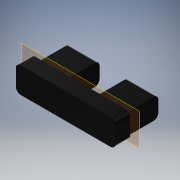
# Autodesk Inventor part: Holster_Button
Saved by Autodesk Inventor 2018 (Build 220112000, 112)
## iProperties
Created: 2018-02-02
Part Number: Holster_Button
Material: Generic
Document SubType Name: Modeling
Designer: Mandus
Density: 1 g/cm^3
Appearance: Default
Author: Mandus
Autodesk Inventor part; units mm, degrees
ref_plane "YZ Plane" through (0, 0, 0) normal (1, 0, 0) x (0, 1, 0)
ref_plane "XZ Plane" through (0, 0, 0) normal (0, 1, 0) x (-1, 0, 0)
ref_plane "XY Plane" through (0, 0, 0) normal (0, 0, 1) x (1, 0, 0)
ref_plane "Work Plane1" through (1.1136, 1.5, 0.2896) normal (0, -1, 0) x (1, 0, 0)
sketch "Sketch3" plane through (1.1136, 1.5, 0.2896) normal (0, -1, 0) x (1, 0, 0)
  line L0 (-8.5, 0) -> (-8.5, 5) construction
  line L1 (-8.5, 5) -> (-1.5, 5) construction
  line L2 (-1.5, 5) -> (-1.5, 0) construction
  line L3 (0, 0) -> (-1.5, 0) construction
  line L4 (0, 0) -> (0, 6) construction
  line L5 (0, 6) -> (-22.065, 6) construction
  line L6 (-22.065, 0) -> (-22.065, 6) construction
  line L7 (-20.565, 0) -> (-22.065, 0) construction
  line L8 (-20.565, 0) -> (-20.565, 5) construction
  line L9 (-20.565, 5) -> (-13.565, 5) construction
  line L10 (-13.565, 5) -> (-13.565, 0) construction
  line L11 (-8.5, 0) -> (-13.565, 0) construction
  line L12 (-0.8, 0) -> (-21.265, 0)
  line L13 (-21.265, 0) -> (-21.265, 5.3)
  line L14 (-21.265, 5.3) -> (-0.8, 5.3)
  line L15 (-0.8, 5.3) -> (-0.8, 0)
  point P0 (-1.1136, -0.2896)
  dimension "d26" = 0.8
  dimension "d27" = 0.8
  dimension "d28" = 0.7
  constraints: 8 end point, 2 parallel, 1 horizontal, 1 perpendicular, 1 point on line
  measures "d26" distance from line of L4 L14.end
  measures "d27" distance from line of L6 L13.end
  measures "d28" distance from line of L5 L13.end
extrude "Extrusion3" add sketch "Sketch3" along normal blind 3
sketch "Sketch4" plane through (1.1136, 1.5, 0.2896) normal (0, 1, 0) x (1, 0, 0)
  line L0 (-8.5, 0) -> (-8.5, -5) construction
  line L1 (-8.5, -5) -> (-1.5, -5) construction
  line L2 (-1.5, -5) -> (-1.5, 0) construction
  line L3 (0, 0) -> (-1.5, 0) construction
  line L4 (0, 0) -> (0, -6) construction
  line L5 (0, -6) -> (-22.065, -6) construction
  line L6 (-22.065, 0) -> (-22.065, -6) construction
  line L7 (-20.565, 0) -> (-22.065, 0) construction
  line L8 (-20.565, 0) -> (-20.565, -5) construction
  line L9 (-20.565, -5) -> (-13.565, -5) construction
  line L10 (-13.565, -5) -> (-13.565, 0) construction
  line L11 (-8.5, 0) -> (-13.565, 0) construction
  line L12 (-2, 0) -> (-8, 0)
  line L13 (-8, 0) -> (-8, -4.3)
  line L14 (-8, -4.3) -> (-2, -4.3)
  line L15 (-2, -4.3) -> (-2, 0)
  line L16 (-0.8, 0) -> (-21.265, 0) projected
  line L17 (-14.065, 0) -> (-20.065, 0)
  line L18 (-20.065, 0) -> (-20.065, -4.3)
  line L19 (-20.065, -4.3) -> (-14.065, -4.3)
  line L20 (-14.065, -4.3) -> (-14.065, 0)
  point P0 (-1.1136, 0.2896)
  point P1 (-5, 0)
  point P2 (-11.0325, 0)
  dimension "d31" = 0.5
  dimension "d32" = 0.5
  dimension "d33" = 0.7
  dimension "d34" = 0.7
  dimension "d35" = 0.5
  dimension "d36" = 0.5
  constraints: 16 end point, 4 parallel, 2 horizontal, 2 midpoint, 2 perpendicular, 1 horizontal alignment, 2 other
  measures "d31" distance from line of L0 L13.end
  measures "d32" distance from line of L2 L14.end
  measures "d33" distance from line of L1 L14.end
  measures "d34" distance from line of L9 L19.end
  measures "d35" distance from line of L10 L19.end
  measures "d36" distance from line of L8 L18.end
extrude "Extrusion4" add sketch "Sketch4" along normal blind 7
fillet "Fillet6" radius 1 4 edges at (-20.1514, 0, 5.5896) (-20.1514, 0, 0.2896) (0.3136, 0, 5.5896) (0.3136, 0, 0.2896)
fillet "Fillet6" radius 1 4 edges at (-3.8864, 8.5, 4.5896) (-3.8864, 8.5, 0.2896) (-15.9514, 8.5, 0.2896) (-15.9514, 8.5, 4.5896)
body "Solid2"
